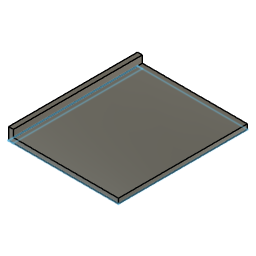
lid (Autodesk Fusion 360 design; units mm, degrees)
Autodesk Fusion 360 part; units mm, degrees
sketch "Sketch1" plane through (0, 0, 0) normal (0, 0, 1) x (1, 0, 0)
  line L0 (0, 50) -> (23, 50)
  line L1 (23, 50) -> (23, 23)
  line L2 (23, 23) -> (0, 23)
  line L3 (0, 23) -> (0, 50)
  line L4 (0, 23) -> (1, 23)
  line L5 (1, 23) -> (1, 50)
  line L6 (1, 50) -> (0, 50)
  line L7 (0, 50) -> (0, 23)
  dimension "d1" = 23
  dimension "d2" = 27
  constraint horizontal L0
  constraint vertical L1
  constraint horizontal L2
  constraint vertical L3
  constraint horizontal L4
  constraint vertical L5
  constraint horizontal L6
  constraint vertical L7
  constraint coincident L0 L5.end
  measures "d1" distance of L0.start L0.end
  measures "d2" distance of L0.start L2.end
extrude "Extrude1" add sketch "Sketch1" along normal blind 1 contours L0 L1 L2 L5
extrude "Extrude2" add sketch "Sketch1" along normal blind 2.5 contours L0 L2 L3 L4 L5 L6 L7
